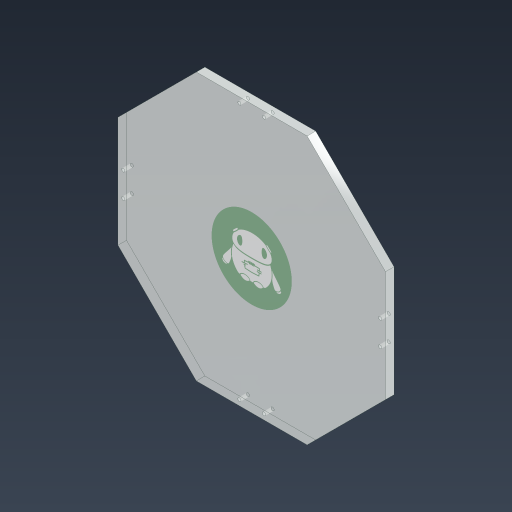
# Autodesk Inventor part: Plate_Acrylic
Saved by Autodesk Inventor 2023 (Build 270158000, 158)
## iProperties
Created: 2024-02-04
Part Number: Plate_Acrylic
Material: Polycarbonate, Clear
Document SubType Name: Modeling
Designer: victo
Density: 1.2 g/cm^3
Appearance: Clear
Author: victo
Autodesk Inventor part; units mm, degrees
ref_plane "YZ Plane" through (0, 0, 0) normal (1, 0, 0) x (0, 1, 0)
ref_plane "XZ Plane" through (0, 0, 0) normal (0, 1, 0) x (-1, 0, 0)
ref_plane "XY Plane" through (0, 0, 0) normal (0, 0, 1) x (1, 0, 0)
sketch "Sketch1" plane through (0, 0, 0) normal (0, 0, 1) x (1, 0, 0)
  line L0 (-51.7767, -125) -> (-125, -51.7767)
  line L1 (-125, -51.7767) -> (-125, 51.7767)
  line L2 (-125, 51.7767) -> (-51.7767, 125)
  line L3 (-51.7767, 125) -> (51.7767, 125)
  line L4 (51.7767, 125) -> (125, 51.7767)
  line L5 (125, 51.7767) -> (125, -51.7767)
  line L6 (125, -51.7767) -> (51.7767, -125)
  line L7 (51.7767, -125) -> (-51.7767, -125)
  circle A0 centre (11.5, -120) radius 1.5
  circle A1 centre (-11.5, -120) radius 1.5
  circle A2 centre (120, 11.5) radius 1.5
  circle A3 centre (120, -11.5) radius 1.5
  circle A4 centre (-11.5, 120) radius 1.5
  circle A5 centre (11.5, 120) radius 1.5
  circle A6 centre (-120, -11.5) radius 1.5
  circle A7 centre (-120, 11.5) radius 1.5
  point P0 (0, 0)
  point P1 (0, 0)
  dimension "d0" = 250
  dimension "d1" = 3
  dimension "d2" = 3
  dimension "d3" = 5
  dimension "d4" = 5
  dimension "d5" = 11.5
  dimension "d6" = 11.5
  dimension "d9" = 360
  constraints: 16 end point, 8 centre point, 1 coincident, 1 horizontal, 34 other
  measures "d0" distance between parallel lines of L3 L7
  measures "d1" diameter of A0
  measures "d2" diameter of A1
  measures "d3" distance from line of L7 A0.centre
  measures "d4" distance from line of L7 A1.centre
  measures "d5" horizontal distance of point (0, 0) A0.centre
  measures "d6" horizontal distance of point (0, 0) A1.centre
extrude "Extrusion1" add sketch "Sketch1" along normal blind 8
sketch "dm" plane through (0, 0, 8) normal (0, 0, 1) x (1, 0, 0)
  line L0 (-37.5, 37.5) -> (37.5, 37.5) construction
  line L1 (37.5, 37.5) -> (37.5, -37.5) construction
  line L2 (37.5, -37.5) -> (-37.5, -37.5) construction
  line L3 (-37.5, -37.5) -> (-37.5, 37.5) construction
  line L4 (-125.8266, 126.5) -> (127.1734, 126.5)
  line L5 (127.1734, 126.5) -> (127.1734, -126.5)
  line L6 (127.1734, -126.5) -> (-125.8266, -126.5)
  line L7 (-125.8266, -126.5) -> (-125.8266, 126.5)
  line L8 (-125.8266, 126.5) -> (127.1734, -126.5) construction
  line L9 (127.1734, 126.5) -> (-125.8266, -126.5) construction
  point P0 (0, 0)
  point P1 (0.6734, 0)
  dimension "d14" = 75
  dimension "d31" = 253
  dimension "d32" = 253
  dimension "d35" = 37.5
  dimension "d36" = 37.5
  dimension "d44" = 37.5
  constraints: 12 end point, 2 midpoint, 2 parallel, 1 horizontal, 1 perpendicular, 2 other
  measures "d14" distance of L2.end L0.start
  measures "d31" distance of L5.end L6.end
  measures "d32" distance of L4.end L5.end
  measures "d35" distance from line of point (0, 0) L1
  measures "d36" distance from line of point (0.673, 0) L2
  measures "d44" distance from line of L0 point (0, 0)
decal "Decal1"
sketch "Sketch3" plane through (0, 0, 8) normal (0, 0, 1) x (1, 0, 0)
  line L0 (51.7767, -125) -> (125, -51.7767) projected
  line L1 (125, -51.7767) -> (125, 51.7767) projected
  line L2 (125, 51.7767) -> (51.7767, 125) projected
  line L3 (51.7767, 125) -> (-51.7767, 125) projected
  line L4 (-51.7767, 125) -> (-125, 51.7767) projected
  line L5 (-125, 51.7767) -> (-125, -51.7767) projected
  line L6 (-125, -51.7767) -> (-51.7767, -125) projected
  line L7 (-51.7767, -125) -> (51.7767, -125) projected
  circle A0 centre (-120, 11.5) radius 1.5 projected
  circle A1 centre (-120, -11.5) radius 1.5 projected
  circle A2 centre (11.5, 120) radius 1.5 projected
  circle A3 centre (-11.5, 120) radius 1.5 projected
  circle A4 centre (120, -11.5) radius 1.5 projected
  circle A5 centre (120, 11.5) radius 1.5 projected
  circle A6 centre (-11.5, -120) radius 1.5 projected
  circle A7 centre (11.5, -120) radius 1.5 projected
  point P0 (0, 0)
equation "\"d4\" = d3"
equation "\"d6\" = d5"
body "Solid1"
